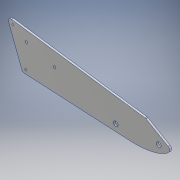
# Autodesk Inventor part: bracket1
Saved by Autodesk Inventor 2018.2 (Build 222227000, 227)
## iProperties
Created: 2018-03-05
Part Number: bracket1
Material: アルミニウム 6061
Document SubType Name: Modeling
Designer: ku_sk
Density: 2.7 g/cm^3
Appearance: アルミニウム - フラット
Mass: 456.161 g
Surface Area: 733.858 cm^2
Volume: 168.949 cm^3
Author: ku_sk
Autodesk Inventor part; units mm, degrees
ref_plane "YZ Plane" through (0, 0, 0) normal (1, 0, 0) x (0, 1, 0)
ref_plane "XZ Plane" through (0, 0, 0) normal (0, 1, 0) x (-1, 0, 0)
ref_plane "XY Plane" through (0, 0, 0) normal (0, 0, 1) x (1, 0, 0)
sketch "スケッチ2" plane through (0, 0, 0) normal (0, 1, 0) x (-1, 0, 0)
  arc A0 (320.7468, 34.8983) -> (392.1215, 71.6787) centre (243.1623, 273.099) ccw projected
  arc A1 (310.5095, 31.8959) -> (320.7468, 34.8983) centre (264.9264, 206.2785) ccw projected
  arc A2 (290.9118, 29.5172) -> (310.5095, 31.8959) centre (291.9468, 102.9093) ccw projected
  arc A3 (278.6891, 31.4878) -> (290.9118, 29.5172) centre (291.5128, 72.1352) ccw projected
  arc A4 (274.9831, 33.389) -> (278.6891, 31.4878) centre (282.4278, 43.3382) ccw projected
  arc A5 (275.4733, 39.2078) -> (274.9831, 33.389) centre (277.0456, 36.1453) ccw projected
  arc A6 (283.1253, 42.3274) -> (275.4733, 39.2078) centre (297.1464, -3.0086) ccw projected
  arc A7 (310.1184, 49.282) -> (283.1253, 42.3274) centre (369.3413, -236.446) ccw projected
  arc A8 (310.1184, 49.282) -> (326.9533, 52.7997) centre (-771.7798, 5269.0252) ccw projected
  arc A9 (326.9533, 52.7997) -> (357.98, 60.8795) centre (256.8539, 385.5961) ccw projected
  arc A10 (357.98, 60.8795) -> (391.1188, 73.3957) centre (268.9975, 346.6028) ccw projected
  arc A11 (392.1215, 71.6787) -> (391.1188, 73.3957) centre (391.5269, 72.4828) ccw projected
  circle A12 centre (287.1934, 37.1564) radius 3 projected
  circle A13 centre (359.7933, 56.2153) radius 3 projected
  arc A14 (100.5026, -29.4375) -> (303.8176, 17.6729) centre (68.6386, 570.3585) ccw projected
  arc A15 (74.9408, -30.0377) -> (100.5026, -29.4375) centre (77.5861, 401.9345) ccw projected
  arc A16 (28.1912, -23.4013) -> (74.9408, -30.0377) centre (76.0159, 145.5175) ccw projected
  arc A17 (1.2395, -11.312) -> (28.1912, -23.4013) centre (55.8939, 74.446) ccw projected
  arc A18 (-6.0217, -4.7376) -> (1.2395, -11.312) centre (16.9451, 13.3315) ccw projected
  arc A19 (-1.6159, 7.4897) -> (-6.0217, -4.7376) centre (0, 0) ccw projected
  arc A20 (17.9572, 9.9554) -> (-1.6159, 7.4897) centre (22.277, -103.2534) ccw projected
  arc A21 (84.7958, 9.311) -> (17.9572, 9.9554) centre (44.6377, -689.2581) ccw projected
  arc A22 (84.7958, 9.311) -> (126.0099, 7.0084) centre (819.0754, 12782.4716) ccw projected
  arc A23 (126.0099, 7.0084) -> (203.0122, 6.466) centre (170.258, 822.6468) ccw projected
  arc A24 (203.0122, 6.466) -> (303.8176, 17.6729) centre (174.1884, 724.7085) ccw projected
  circle A25 centre (20.0666, -1.5588) radius 5 projected
  circle A26 centre (130.4331, -10.1322) radius 5 projected
  line L0 (100.5026, -29.4375) -> (370, -15.1205)
  line L1 (-3.831, 6.6355) -> (54.1787, 40.1274)
  line L2 (1137.2465, 0) -> (-1089.9509, 0) projected
  line L3 (54.1787, 40.1274) -> (410, 89.8795)
  line L4 (370, -15.1205) -> (410, 89.8795)
  point P0 (0, 0)
  point P1 (371.2778, 57.8193)
  dimension "d7" = 30
  dimension "d115" = 370
  dimension "d164" = 40
  dimension "d165" = 105
  constraints: 8 end point, 2 point on circle, 2 tangent
  measures "d7" angle of L2 L1
  measures "d115" horizontal distance of L0.end point (0, 0)
  measures "d164" horizontal distance of L3.end L0.end
  measures "d165" vertical distance of L0.end L3.end
extrude "押し出し3" add sketch "スケッチ2" along normal blind 5 contours A1 A2 A3 A4 A5 A6 A7 A8 A9 A10 A11 A0 | A15 A16 A17 A18 A19 L2 A25 A14 | A14 L2 L4 L0 | L2 A25 A19 A20 A21 A22 A23 A24 A14 | A14 A24 A23 A22 A21 A20 A19 L1 L3 L4 L2
fillet "フィレット2" radius 6 2 edges at (-54.1787, 2.5, 40.1274) (-370, 2.5, -15.1205)
fillet "フィレット2" radius 7 1 edges at (-410, 2.5, 89.8795)
sketch "スケッチ4" plane through (0, 5, 0) normal (0, 1, 0) x (1, 0, 0)
  circle A0 centre (-361.3333, 5.5668) radius 2.5
  line L0 (-53.1667, -39.5431) -> (3.831, -6.6355) projected
  line L1 (-410, -89.8795) -> (-55.3359, -40.2892) projected
  line L2 (-100.5026, 29.4375) -> (-366.1013, 15.3276) projected
  line L3 (-371.3899, 11.472) -> (-410, -89.8795) projected
  circle A1 centre (-394.6339, -77.6337) radius 2.5
  point P0 (0, 0)
  dimension "d21" = 5
  dimension "d22" = 10
  dimension "d23" = 11.5
  dimension "d77" = 10
  dimension "d78" = 10
  dimension "d79" = 5
  constraints: 2 centre point
  measures "d21" diameter of A0
  measures "d22" distance from line of L2 A0.centre
  measures "d23" distance from line of L3 A0.centre
  measures "d77" distance from line of A1.centre L1
  measures "d78" distance from line of L3 A1.centre
  measures "d79" diameter of A1
sketch "スケッチ6" plane through (0, 0, 0) normal (0, -1, 0) x (1, 0, 0)
  circle A0 centre (-20.0666, -1.5588) radius 6
  circle A1 centre (-20.0666, -1.5588) radius 5 projected
  circle A2 centre (-130.4331, -10.1322) radius 6
  circle A3 centre (-130.4331, -10.1322) radius 5 projected
  point P0 (0, 0)
  dimension "d29" = 12
  dimension "d30" = 12
  constraints: 2 centre point, 2 concentric
  measures "d29" diameter of A0
  measures "d30" diameter of A2
extrude "押し出し7" cut sketch "スケッチ6" against normal through all
extrude "押し出し9" cut sketch "スケッチ4" against normal through all
